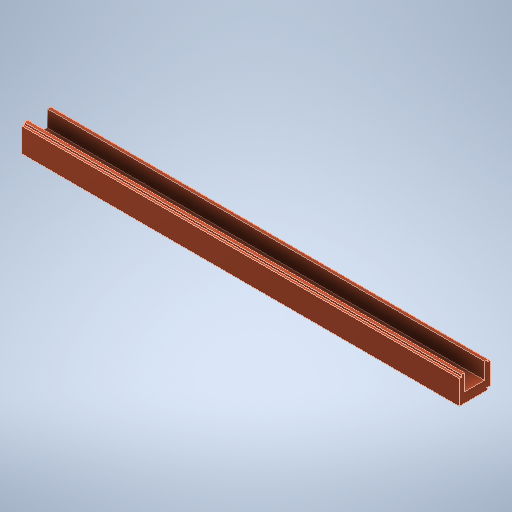
# Autodesk Inventor part: Zarge
Saved by Autodesk Inventor 2025.1 (Build 291241000, 241)
## iProperties
Created: 2024-08-07
Part Number: Zarge
Material: Copper
Document SubType Name: Modeling
Designer: ffogue
Density: 8.94 g/cm^3
Appearance: Copper - Satin
Author: ffogue
Autodesk Inventor part; units mm, degrees
ref_plane "YZ Plane" through (0, 0, 0) normal (1, 0, 0) x (0, 1, 0)
ref_plane "XZ Plane" through (0, 0, 0) normal (0, 1, 0) x (-1, 0, 0)
ref_plane "XY Plane" through (0, 0, 0) normal (0, 0, 1) x (1, 0, 0)
sketch "Sketch1" plane through (0, 0, 0) normal (1, 0, 0) x (0, 1, 0)
  line L0 (70, 0) -> (-70, 0)
  line L1 (-70, 0) -> (-70, 100)
  line L2 (-70, 100) -> (-60, 100)
  line L3 (-60, 100) -> (-60, 110)
  line L4 (-60, 110) -> (-45, 110)
  line L5 (-45, 110) -> (-45, 95)
  line L6 (-45, 95) -> (-45, 95)
  line L7 (-45, 95) -> (-45, 35)
  line L8 (-45, 35) -> (45, 35)
  line L9 (45, 35) -> (45, 95)
  line L10 (45, 95) -> (45, 95)
  line L11 (45, 95) -> (45, 110)
  line L12 (45, 110) -> (60, 110)
  line L13 (60, 110) -> (60, 100)
  line L14 (60, 100) -> (70, 100)
  line L15 (70, 100) -> (70, 0)
  point P0 (0, 0)
  point P1 (0, 0)
  point P2 (0, 35)
  dimension "d15" = 90
  dimension "d16" = 110
  dimension "d17" = 10
  dimension "d20" = 35
  dimension "d21" = 15
  dimension "d22" = 15
  dimension "d23" = 15
  dimension "d24" = 10
  dimension "d25" = 10
  dimension "d26" = 135
  dimension "d27" = 135
  dimension "d28" = 90
  constraints: 32 end point, 8 perpendicular, 4 point on line, 3 parallel, 2 midpoint, 1 coincident, 1 horizontal, 1 horizontal alignment, 1 vertical alignment
  measures "d15" distance between parallel lines of L5 L11
  measures "d16" distance between parallel lines of L0 L12
  measures "d17" distance of L12.end L13.end
  measures "d20" distance between parallel lines of L0 L8
  measures "d21" distance of L10.end L11.end
  measures "d22" distance of L4.end L5.end
  measures "d23" distance of L11.end L12.end
  measures "d24" distance between parallel lines of L1 L3
  measures "d25" distance of L13.end L14.end
  measures "d26" angle of L9 L10
  measures "d27" angle of L7 L6
  measures "d28" distance of L7.end L8.end
extrude "Extrusion1" add sketch "Sketch1" against normal blind 1985
sketch "Sketch2" plane through (0, 0, 0) normal (1, 0, 0) x (0, 0, -1)
  line L0 (0, -70) -> (0, 70) projected
  line L1 (-110, 45) -> (-35, 45) projected
  line L2 (0, 25) -> (0, 45)
  line L3 (0, 70) -> (0, -70) projected
  line L4 (0, -70) -> (10, -70)
  line L5 (0, 55) -> (10, 55)
  line L6 (10, 55) -> (10, -70)
  line L7 (5, 55) -> (5, 30.8047) construction
  line L8 (0, 70) -> (-100, 70) projected
  line L9 (10, 55) -> (5, 70)
  line L10 (5, 70) -> (0, 55)
  point P0 (0, 0)
  point P1 (5, -70)
  point P2 (0, 55)
  dimension "d36" = 10
  dimension "d43" = 15
  constraints: 14 end point, 3 point on line, 2 midpoint, 2 vertical, 2 vertical alignment, 1 horizontal alignment, 1 perpendicular, 1 symmetric about line
  measures "d36" distance of L4.start L4.end
  measures "d43" distance from line of L7.start L8
extrude "Extrusion2" add sketch "Sketch2" against normal up to surface (1985 mm away)
fillet "Fillet2" radius 5 1 edges at (-992.5, 70, -5)
equation "\"d22\" = d21"
equation "\"d25\" = d17"
body "Solid1"
